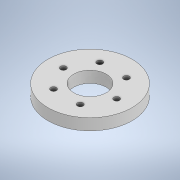
# Autodesk Inventor part: driving system S4
Saved by Autodesk Inventor 2022.2 (Build 262287000, 287)
## iProperties
Created: 2022-03-05
Part Number: driving system S4
Material: Generic
Document SubType Name: Modeling
Designer: zyao2
Density: 1 g/cm^3
Appearance: Default
Author: zyao2
Autodesk Inventor part; units mm, degrees
ref_plane "YZ Plane" through (0, 0, 0) normal (1, 0, 0) x (0, 1, 0)
ref_plane "XZ Plane" through (0, 0, 0) normal (0, 1, 0) x (-1, 0, 0)
ref_plane "XY Plane" through (0, 0, 0) normal (0, 0, 1) x (1, 0, 0)
sketch "Sketch1" plane through (0, 0, 0) normal (0, 1, 0) x (-1, 0, 0)
  circle A0 centre (0, 0) radius 37.5
  circle A1 centre (0, 0) radius 14.5
  line L0 (0, 0) -> (23.813, 0)
  circle A2 centre (23.813, 0) radius 2.56
  circle A3 centre (11.9065, 20.6227) radius 2.56
  circle A4 centre (-11.9065, 20.6227) radius 2.56
  circle A5 centre (-23.813, 0) radius 2.56
  circle A6 centre (-11.9065, -20.6227) radius 2.56
  circle A7 centre (11.9065, -20.6227) radius 2.56
  dimension "d0" = 75
  dimension "d1" = 29
  dimension "d2" = 23.813
  dimension "d3" = 5.12
  dimension "d6" = 360
  constraints: 8 centre point, 3 coincident, 2 end point, 1 horizontal, 13 other
  measures "d0" diameter of A0
  measures "d1" diameter of A1
  measures "d2" distance of L0.start L0.end
  measures "d3" diameter of A2
extrude "Extrusion1" add sketch "Sketch1" along normal blind 10.16
body "Solid1"
